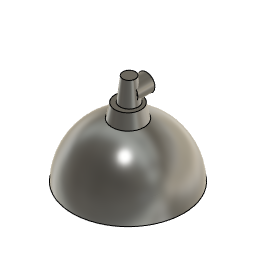
oho v4 (Autodesk Fusion 360 design; units mm, degrees)
Autodesk Fusion 360 part; units mm, degrees
note: some values were not read from the file. Set by a fixed rule: which sketch regions a step uses.
sketch "Sketch3" plane through (0, 0, 0) normal (0, 1, 0) x (1, 0, 0)
  line L0 (0, -100) -> (30, -100)
  line L1 (24.5205, -124.6096) -> (30, -100)
  line L2 (24.5205, -124.6096) -> (0, -124.6096)
  arc A0 (30, -100) -> (100, 0) centre (-8.0769, 1.1538) ccw
  line L3 (100, 0) -> (0, 0)
  line L4 (2, -2) -> (2, -122.6096)
  line L5 (97.9593, -2) -> (2, -2)
  arc A1 (28.2844, -98.503) -> (97.9593, -2) centre (-8.0769, 1.1538) ccw
  line L6 (22.9168, -122.6096) -> (28.2844, -98.503)
  line L7 (22.9168, -122.6096) -> (2, -122.6096)
  line L8 (26.1241, -126.6096) -> (0, -126.6096)
  line L9 (26.1241, -126.6096) -> (31.9522, -100.4347)
  line L10 (18.1129, -126.6096) -> (13.0621, -166.7452)
  line L11 (13.0621, -166.7452) -> (2, -166.7452)
  line L12 (2, -166.7452) -> (2, -124.6096)
  dimension "d8" = -2
  constraint horizontal L0
  constraint parallel L0 L2
  constraint coincident L3.end origin
  constraint horizontal L3
  constraint parallel L3 L5
  constraint concentric A0 A1
  constraint parallel L1 L6
  constraint parallel L2 L7
  constraint coincident L8 L10.start
  constraint perpendicular L4 L11
  constraint perpendicular L8 L12
revolve "Revolve1" add sketch "Sketch3" angle 360 about axis through (0, 0, 0) along (0, 0, 1) contours L0 L4 L5 A1 L6 makes body 1
revolve "Revolve2" add sketch "Sketch3" angle 360 about axis through (0, 0, 0) along (0, 0, 1) contours L0 L4 L6 L7 bodies 1
revolve "Revolve3" add sketch "Sketch3" angle 360 about axis through (2, 0, 2) along (0, 0, 1) separate body contours L8 L10 L11 L12 makes body 2
move_body "Move1" bodies 2 to x (1, 0, 0) y (0, 1, 0) z (0, 0, 1) at (0, 0, -2)
sketch "Sketch4" plane through (0, 0, 0) normal (0, 1, 0) x (1, 0, 0)
  circle A0 centre (0, -150) radius 15
  circle A1 centre (0, -150) radius 13
  dimension "d13" = 30
  dimension "d14" = 26
  constraint concentric A0 A1
  measures "d13" diameter of A0
  measures "d14" diameter of A1
extrude "Extrude1" add sketch "Sketch4" along normal blind 30 separate body makes body 3
move_body "Move2" bodies 3 to x (1, 0, 0) y (0, 1, 0) z (0, 0, 1) at (0, 0, -20)
move_body "Move3" bodies 3 to x (1, 0, 0) y (0, 1, 0) z (0, 0, 1) at (0, 0, 10)
move_body "Move4" bodies 3 to x (1, 0, 0) y (0, 1, 0) z (0, 0, 1) at (0.2, 0, 0)
move_body "Move5" bodies 3 to x (1, 0, 0) y (0, 1, 0) z (0, 0, 1) at (0.2, 0, 0)
move_body "Move6" bodies 3 to x (1, 0, 0) y (0, 1, 0) z (0, 0, 1) at (2, 0, 0)
